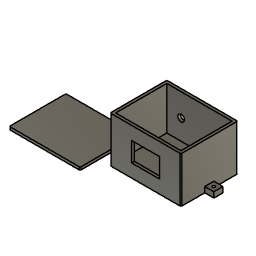
Box and lid v4 (Autodesk Fusion 360 design; units mm, degrees)
Autodesk Fusion 360 part; units mm, degrees
note: some values were not read from the file. Chosen so that the rebuilt part matches the saved one: which bodies a step acts on.
sketch "Sketch4" plane through (0, 0, 0) normal (0, 0, 1) x (1, 0, 0)
  line L0 (38.75, -31) -> (-38.75, -31)
  line L1 (-38.75, -31) -> (-38.75, 31)
  line L2 (-38.75, 31) -> (38.75, 31)
  line L3 (38.75, 31) -> (38.75, -31)
  line L4 (38.75, -31) -> (-38.75, 31) construction
  line L5 (-38.75, -31) -> (38.75, 31) construction
  dimension "d14" = 77.5
  dimension "d15" = 62
  constraint horizontal L0
  constraint perpendicular L0 L1
  constraint parallel L0 L2
  constraint parallel L1 L3
  constraint coincident L4 origin
  constraint coincident L5 origin
  measures "d14" distance of L1 L3
  measures "d15" distance of L0 L2
extrude "Extrude4" add sketch "Sketch4" along normal blind 50 makes body 1
sketch "Sketch5" plane through (0, 0, 50) normal (0, 0, 1) x (-1, 0, 0)
  line L0 (-38.75, -31) -> (38.75, -31)
  line L1 (38.75, -31) -> (38.75, 31)
  line L2 (38.75, 31) -> (-38.75, 31)
  line L3 (-38.75, 31) -> (-38.75, -31)
  line L4 (-35.75, 28) -> (35.75, 28)
  line L5 (35.75, 28) -> (35.75, -28)
  line L6 (35.75, -28) -> (-35.75, -28)
  line L7 (-35.75, -28) -> (-35.75, 28)
  line L8 (-35.75, 28) -> (35.75, -28) construction
  line L9 (35.75, 28) -> (-35.75, -28) construction
  dimension "d18" = 71.5
  dimension "d19" = 56
  constraint horizontal L4
  constraint perpendicular L4 L5
  constraint parallel L4 L6
  constraint parallel L5 L7
  constraint coincident L8 origin
  constraint coincident L9 origin
  measures "d18" distance of L5 L7
  measures "d19" distance of L4 L6
extrude "Extrude5" cut sketch "Sketch5" against normal blind 47 contours L4 L5 L6 L7 bodies 1
sketch "Sketch6" plane through (0, -31, 0) normal (0, -1, 0) x (1, 0, 0)
  line L0 (-38.75, 0) -> (38.75, 0)
  line L1 (38.75, 0) -> (38.75, 50)
  line L2 (38.75, 50) -> (-38.75, 50)
  line L3 (-38.75, 50) -> (-38.75, 0)
  line L4 (15.3, 14.375) -> (-15.3, 14.375)
  line L5 (-15.3, 14.375) -> (-15.3, 35.625)
  line L6 (-15.3, 35.625) -> (15.3, 35.625)
  line L7 (15.3, 35.625) -> (15.3, 14.375)
  line L8 (15.3, 14.375) -> (-15.3, 35.625) construction
  line L9 (-15.3, 14.375) -> (15.3, 35.625) construction
  point P0 (0, 25)
  dimension "d22" = 30.6
  dimension "d23" = 21.25
  constraint horizontal L4
  constraint perpendicular L4 L5
  constraint parallel L4 L6
  constraint parallel L5 L7
  constraint coincident L8 P0
  constraint coincident L9 P0
  measures "d22" distance of L5 L7
  measures "d23" distance of L4 L6
extrude "Extrude6" cut sketch "Sketch6" against normal blind 5 contours L4 L5 L6 L7 bodies 1
sketch "Sketch7" plane through (0, 31, 0) normal (0, 1, 0) x (-1, 0, 0)
  line L0 (-38.75, 0) -> (38.75, 0)
  line L1 (38.75, 0) -> (38.75, 50)
  line L2 (38.75, 50) -> (-38.75, 50)
  line L3 (-38.75, 50) -> (-38.75, 0)
  line L4 (0, 60) -> (0, -15)
  circle A0 centre (-20, 25) radius 3.675
  circle A1 centre (20, 25) radius 3.675
  dimension "d26" = 7.35
  dimension "d27" = 7.35
  constraint perpendicular L0 L4
  measures "d26" diameter of A0
  measures "d27" diameter of A1
extrude "Extrude7" cut sketch "Sketch7" against normal blind 5 contours A0 bodies 1
extrude "Extrude8" cut sketch "Sketch7" against normal blind 5 contours A1 bodies 1
sketch "Sketch8" plane through (0, 0, 3) normal (0, 0, 1) x (-1, 0, 0)
  line L0 (-35.75, -28) -> (35.75, -28)
  line L1 (35.75, -28) -> (35.75, 28)
  line L2 (35.75, 28) -> (-35.75, 28)
  line L3 (-35.75, 28) -> (-35.75, -28)
  line L4 (49, -5) -> (39, -5)
  line L5 (39, -5) -> (39, 5)
  line L6 (39, 5) -> (49, 5)
  line L7 (49, 5) -> (49, -5)
  dimension "d32" = 10
  dimension "d33" = 10
  constraint horizontal L4
  constraint vertical L5
  constraint horizontal L6
  constraint vertical L7
  measures "d32" distance of L5 L7
  measures "d33" distance of L4 L6
extrude "Extrude9" add sketch "Sketch8" along normal blind 6 separate body contours L4 L5 L6 L7 makes body 2
move_body "Move1" bodies 2 to x (1, 0, 0) y (0, 1, 0) z (0, 0, 1) at (0, 0, -3)
sketch "Sketch9" plane through (0, 0, 3) normal (0, 0, 1) x (1, 0, 0)
move_body "Move2" bodies 2 to x (1, 0, 0) y (0, 1, 0) z (0, 0, 1) at (0.2552, 0.0123, 0.0295)
copy_body "CopyPasteBodies1" bodies 2 makes body 3
move_body "Move6" bodies 3 to x (1, 0, 0) y (0, 1, 0) z (0, 0, 1) at (93.1162, 1.1461, -0.8039)
move_body "Move7" bodies 3 to x (1, 0, 0) y (0, 1, 0) z (0, 0, 1) at (-5.6154, -0.0546, 0.8185)
move_body "Move8" bodies 3 to x (1, 0, 0) y (0, 1, 0) z (0, 0, 1) at (-0.001, -0.0016, -0.035)
move_body "Move9" bodies 3 to x (1, 0, 0) y (0, 1, 0) z (0, 0, 1) at (-0.0011, 0, -0.0074)
move_body "Move10" bodies 3 to x (1, 0, 0) y (0, 1, 0) z (0, 0, 1) at (0.0091, 0.0008, -0.0049)
move_body "Move11" bodies 3 to x (1, 0, 0) y (0, 1, 0) z (0, 0, 1) at (0.0747, -1.0616, 0.0059)
sketch "Sketch14" plane through (0, 0, 6.0295) normal (0, 0, 1) x (-1, 0, 0)
  line L0 (48.7448, 4.9877) -> (38.7448, 4.9877)
  line L1 (38.7448, 4.9877) -> (38.7448, -5.0123)
  line L2 (38.7448, -5.0123) -> (48.7448, -5.0123)
  line L3 (48.7448, -5.0123) -> (48.7448, 4.9877)
combine "Combine2" operation add target body 1 tool bodies 3 2 makes body 4 at (45.5043, 1.7081, 0.0028)
sketch "Sketch15" plane through (0, 0, 6.0295) normal (0, 0, 1) x (-1, 0, 0)
  circle A0 centre (43.766, 0.0007) radius 1.5
  dimension "d51" = 3
  measures "d51" diameter of A0
extrude "Extrude13" cut sketch "Sketch15" against normal blind 7 bodies 1
sketch "Sketch16" plane through (0, 0, 6.0028) normal (0, 0, 1) x (-1, 0, 0)
  line L0 (-38.8377, 4.9586) -> (-48.8377, 4.9586)
  line L1 (-48.8377, 4.9586) -> (-48.8377, -5.0414)
  line L2 (-48.8377, -5.0414) -> (-38.8377, -5.0414)
  line L3 (-38.8377, -5.0414) -> (-38.8377, 4.9586)
  circle A0 centre (-43.9, 0) radius 1.5
  dimension "d54" = 3
  measures "d54" diameter of A0
extrude "Extrude14" cut sketch "Sketch16" against normal blind 6 contours A0 bodies 4
combine "Combine3" operation add target body 1 tool bodies 4 makes body 5 at (40.0251, 0.0276, 0.0028)
combine "Combine4" operation add target body 1 tool bodies 5 makes body 6 at (40.0251, 0.0276, 0.0028)
move_body "Move13" bodies 6 to x (1, 0, 0) y (0, 1, 0) z (0, 0, 1) at (-0.09, 0, 0)
combine "Combine5" operation add target body 6 tool bodies 1
fillet "Fillet3" radius 1 4 edges at (-38.75, 31, 25) (-38.75, -31, 25) (38.75, 31, 25) (38.75, -31, 25) on bodies 6
sketch "Sketch17" plane through (0, 0, 3) normal (0, 0, 1) x (-1, 0, 0)
  line L0 (-35.75, -28) -> (35.75, -28)
  line L1 (35.75, -28) -> (35.75, 28)
  line L2 (35.75, 28) -> (-35.75, 28)
  line L3 (-35.75, 28) -> (-35.75, -28)
  line L4 (130.2279, -12.0353) -> (52.7279, -12.0353)
  line L5 (52.7279, -12.0353) -> (52.7279, 49.9647)
  line L6 (52.7279, 49.9647) -> (130.2279, 49.9647)
  line L7 (130.2279, 49.9647) -> (130.2279, -12.0353)
  dimension "d59" = 62
  dimension "d60" = 77.5
  constraint horizontal L4
  constraint vertical L5
  constraint horizontal L6
  constraint vertical L7
  measures "d59" distance of L4 L6
  measures "d60" distance of L5 L7
extrude "Extrude15" add sketch "Sketch17" along normal blind 3 separate body contours L4 L5 L6 L7 makes body 7
move_body "Move14" bodies 7 to x (1, 0, 0) y (0, 1, 0) z (0, 0, 1) at (0, 0, -5)
fillet "Fillet4" radius 1 4 edges at (-52.7279, -49.9647, -0.5) (-52.7279, 12.0353, -0.5) (-130.2279, -49.9647, -0.5) (-130.2279, 12.0353, -0.5) on bodies 7
move_body "Move3" [suppressed]
sketch "Sketch10" plane through (0, 0, 6.0295) normal (0, 0, 1) x (-1, 0, 0)
  line L0 (48.7448, 4.9877) -> (38.7448, 4.9877)
  line L1 (38.7448, 4.9877) -> (38.7448, -5.0123)
  line L2 (38.7448, -5.0123) -> (48.7448, -5.0123)
  line L3 (48.7448, -5.0123) -> (48.7448, 4.9877)
  circle A0 centre (43.5, 0) radius 1.825
  circle A1 centre (43.5, 0) radius 1.825
  point P0 (-43.5043, -0.185)
  point P1 (43.5, 0)
  dimension "d36" = 3.65
  dimension "d37" = 3.65
  constraint coincident P1 A0.centre
  measures "d36" diameter of A0
  measures "d37" diameter of A1
extrude "Extrude10" [suppressed]
sketch "Sketch11" plane through (0, 0, 6.2043) normal (0, 0, 1) x (-1, 0, 0)
  line L0 (-136.3262, -4.9957) -> (-126.3262, -4.9957)
  line L1 (-126.3262, -4.9957) -> (-126.3262, 5.0043)
  line L2 (-126.3262, 5.0043) -> (-136.3262, 5.0043)
  line L3 (-136.3262, 5.0043) -> (-136.3262, -4.9957)
  circle A0 centre (-43.4472, -0.0093) radius 1.825
  dimension "d40" = 3.65
  measures "d40" diameter of A0
extrude "Extrude11" [suppressed]
combine "Combine1" [suppressed]
sketch "Sketch13" plane through (0, 0, 50) normal (0, 0, 1) x (-1, 0, 0)
  line L0 (35.75, 28) -> (35.75, -28)
  line L1 (35.75, -28) -> (-35.75, -28)
  line L2 (-35.75, -28) -> (-35.75, 28)
  line L3 (-35.75, 28) -> (35.75, 28)
  line L4 (-38.75, -31) -> (38.75, -31)
  line L5 (38.75, -31) -> (38.75, 31)
  line L6 (38.75, 31) -> (-38.75, 31)
  line L7 (-38.75, 31) -> (-38.75, -31)
  line L8 (125.1983, 10) -> (47.6983, 10)
  line L9 (47.6983, 10) -> (47.6983, 72)
  line L10 (47.6983, 72) -> (125.1983, 72)
  line L11 (125.1983, 72) -> (125.1983, 10)
  dimension "d43" = 62
  dimension "d44" = 77.5
  constraint horizontal L8
  constraint vertical L9
  constraint horizontal L10
  constraint vertical L11
  measures "d43" distance of L8 L10
  measures "d44" distance of L9 L11
extrude "Extrude12" [suppressed]
move_body "Move4" [suppressed]
move_body "Move5" [suppressed]
fillet "Fillet1" [suppressed]
fillet "Fillet2" [suppressed]
extrude "Extrude1" [suppressed]
sketch "Sketch2" plane through (0, 0, 50) normal (0, 0, 1) x (-1, 0, 0)
  line L0 (22.5, 37) -> (-55, 37)
  line L1 (-55, 37) -> (-55, -25)
  line L2 (-55, -25) -> (22.5, -25)
  line L3 (22.5, -25) -> (22.5, 37)
  line L4 (-51.3638, 33.3638) -> (-51.3638, -21.3638)
  line L5 (-51.3638, -21.3638) -> (18.8638, -21.3638)
  line L6 (18.8638, -21.3638) -> (18.8638, 33.3638)
  line L7 (18.8638, 33.3638) -> (-51.3638, 33.3638)
  dimension "d7" = -3.6362
extrude "Extrude2" [suppressed]
extrude "Extrude3" [suppressed]
sketch "Sketch3" plane through (0, -37, 0) normal (0, -1, 0) x (1, 0, 0)
  line L0 (-22.5, 0) -> (55, 0)
  line L1 (55, 0) -> (55, 50)
  line L2 (55, 50) -> (-22.5, 50)
  line L3 (-22.5, 50) -> (-22.5, 0)
  line L4 (1.8537, 36.4577) -> (32.4537, 36.4577)
  line L5 (32.4537, 36.4577) -> (32.4537, 11.7577)
  line L6 (32.4537, 11.7577) -> (1.8537, 11.7577)
  line L7 (1.8537, 11.7577) -> (1.8537, 36.4577)
  dimension "d12" = 24.7
  dimension "d13" = 30.6
  constraint horizontal L4
  constraint vertical L5
  constraint horizontal L6
  constraint vertical L7
  measures "d12" distance of L4 L6
  measures "d13" distance of L5 L7
move_body "Move12" [suppressed]
